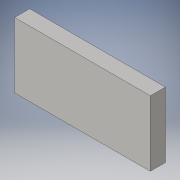
# Autodesk Inventor part: cwbattery
Saved by Autodesk Inventor 2016 (Build 200138000, 138)
## iProperties
Created: 2017-09-05
Part Number: cwbattery
Material: Generic
Document SubType Name: Modeling
Designer: student
Density: 1 g/cm^3
Appearance: Default
Author: student
Autodesk Inventor part; units mm, degrees
ref_plane "YZ Plane" through (0, 0, 0) normal (1, 0, 0) x (0, 1, 0)
ref_plane "XZ Plane" through (0, 0, 0) normal (0, 1, 0) x (-1, 0, 0)
ref_plane "XY Plane" through (0, 0, 0) normal (0, 0, 1) x (1, 0, 0)
sketch "Sketch1" plane through (0, 0, 0) normal (0, 0, 1) x (1, 0, 0)
  line L0 (-34.29, -16.51) -> (34.29, -16.51)
  line L1 (34.29, -16.51) -> (34.29, 16.51)
  line L2 (34.29, 16.51) -> (-34.29, 16.51)
  line L3 (-34.29, 16.51) -> (-34.29, -16.51)
  point P0 (0, 0)
  dimension "d0" = 68.58
  dimension "d1" = 33.02
  constraints: 8 end point, 2 parallel, 1 horizontal, 1 perpendicular
  measures "d0" distance of L1.end L2.end
  measures "d1" distance of L0.end L1.end
extrude "Extrusion1" add sketch "Sketch1" along normal blind 7.62
body "Solid1"
